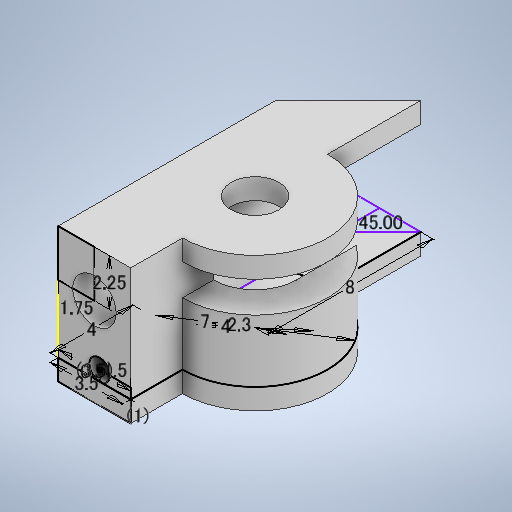
# Autodesk Inventor part: rod6.0
Saved by Autodesk Inventor 2025 (Build 290162000, 162)
## iProperties
Created: 2024-08-07
Part Number: rod6.0
Material: 一般
Document SubType Name: Modeling
Designer: Saigusa
Density: 1 g/cm^3
Appearance: 既定
Author: Saigusa
Autodesk Inventor part; units mm, degrees
ref_plane "YZ Plane" through (0, 0, 0) normal (1, 0, 0) x (0, 1, 0)
ref_plane "XZ Plane" through (0, 0, 0) normal (0, 1, 0) x (-1, 0, 0)
ref_plane "XY Plane" through (0, 0, 0) normal (0, 0, 1) x (1, 0, 0)
sketch "スケッチ1" plane through (0, 0, 0) normal (0, 1, 0) x (-1, 0, 0)
  circle A0 centre (0, 0) radius 1.15
  circle A1 centre (0, 0) radius 2
  circle A2 centre (0, 0) radius 3.5
  line L0 (0, 0) -> (0, 3.5)
  line L1 (2, 0) -> (-2, 0)
  line L2 (2, 0) -> (2, -2.8723)
  line L3 (-2, 0) -> (-2, -2.8723)
  line L4 (0, 2) -> (3.5, 2)
  line L5 (3.5, 2) -> (3.5, 6)
  line L6 (3.5, 6) -> (0, 6)
  line L7 (0, 6) -> (0, 2)
  line L8 (0, 6) -> (3.5, 6)
  line L9 (3.5, 6) -> (3.5, 0)
  line L10 (3.5, 0) -> (0, 0)
  line L11 (0, 0) -> (0, 6)
  line L12 (0, 0) -> (0, -8)
  line L13 (0, 0) -> (3.5, 0)
  line L14 (3.5, 0) -> (3.5, -8)
  line L15 (3.5, -8) -> (0, -8)
  line L16 (0, -8) -> (0, 0)
  line L17 (2, -2.8723) -> (2, -8)
  line L18 (0, -8) -> (3.5, -4.5)
  line L19 (0, -8) -> (4.9497, -8) construction
  point P0 (2, -6)
  point P1 (0, -3.5)
  dimension "d0" = 2.3
  dimension "d1" = 4
  dimension "d2" = 7
  dimension "d3" = 3.5
  dimension "d4" = 4
  dimension "d5" = 8
  dimension "d6" = 45
  constraints: 40 end point, 7 perpendicular, 7 point on circle, 6 parallel, 4 horizontal, 3 centre point, 3 coincident, 3 point on line, 2 vertical, 1 equal length
  measures "d0" diameter of A0
  measures "d1" diameter of A1
  measures "d2" diameter of A2
  measures "d3" distance of L6.end L5.end
  measures "d4" distance of L5.end L4.end
  measures "d5" distance of L10.end L12.end
  measures "d6" angle of L19 L18
extrude "押し出し1" add sketch "スケッチ1" along normal blind 3 contours A1 L3 A2 L0
extrude "押し出し2" add sketch "スケッチ1" along normal blind 4.5 contours L10 A2 L2 | A1 L4 A2 L10 | L0 A2 L4 | A2 L14 L18 L17 | A2 L4 L9 | L7 L6 L5 L4 A2
extrude "押し出し3" add sketch "スケッチ1" against normal blind 1 contours L1 A1 L12 A0 | A0 L0 A1 L1 | A0 L1 A1 L0 | L12 A1 L1 A0 | L2 A2 L12 A1 | L10 A2 L2 | A1 L4 A2 L10 | A1 L3 A2 L0 | L0 A2 L4 | L12 A2 L3 A1 | L17 L18 L12 A2 | A2 L14 L18 L17 | A2 L4 L9 | L7 L6 L5 L4 A2
sketch "スケッチ2" plane through (0, 4.5, 0) normal (0, 1, 0) x (1, 0, 0)
  circle A0 centre (0, 0) radius 1.15
  circle A1 centre (0, 0) radius 2
  circle A2 centre (0, 0) radius 3.5
  line L0 (0, -2) -> (0, -3.5) projected
  line L1 (-3.5, 4.5) -> (-3.5, -6) projected
  line L2 (0, -2) -> (-3.5, -2)
  line L3 (-3.5, -2) -> (-3.5, -6)
  line L4 (-3.5, -6) -> (0, -6)
  line L5 (0, -6) -> (0, -2)
  line L6 (0, -2) -> (-3.5, -2)
  line L7 (-3.5, -2) -> (-3.5, 8)
  line L8 (-3.5, 8) -> (0, 8)
  line L9 (0, 8) -> (0, -2)
  line L10 (0, 0) -> (-2, 0)
  line L11 (-2, 0) -> (-2, 8)
  line L12 (-2, 8) -> (0, 8)
  line L13 (0, 8) -> (0, 0)
  line L14 (0, 8) -> (-3.5, 4.5)
  line L15 (0, 8) -> (4.9497, 8) construction
  point P0 (0, 3.5)
  dimension "d14" = 4
  dimension "d15" = 7
  dimension "d13" = 2.3
  dimension "d16" = 3.5
  dimension "d17" = 4
  dimension "d18" = 3.5
  dimension "d19" = 10
  dimension "d20" = 2
  dimension "d21" = 8
  dimension "d22" = 135
  constraints: 28 end point, 6 parallel, 4 horizontal, 3 coincident, 3 perpendicular, 1 centre point, 1 equal length, 1 vertical alignment, 3 other
  measures "d13" diameter of A0
  measures "d16" distance of L4.end L1.end
  measures "d17" distance of L1.end L2.end
  measures "d18" distance of L7.end L8.end
  measures "d19" distance of L6.end L7.end
  measures "d20" distance of L11.end L12.end
  measures "d21" distance of L10.end L11.end
  measures "d22" angle of L14 L15
extrude "押し出し4" add sketch "スケッチ2" along normal blind 1 contours A0 L9 A1 | A0 L10 A1 L9 | L9 A1 L10 A0 | L9 A2 L0 A1 | A1 L11 A2 L9 | L2 A2 L11 A1 | L0 A2 L2 | A2 L11 L14 L9 | L5 L4 L1 L2 A2 | L2 L1 A2 | A2 L1 L14 L11
sketch "スケッチ3" plane through (-3.5, -1, 6) normal (0, 0, 1) x (1, 0, 0)
  line L0 (0, 0) -> (0, 6.5) projected
  line L1 (0, 0) -> (3.5, 0)
  line L2 (3.5, 0) -> (3.5, 1)
  line L3 (3.5, 1) -> (0, 1)
  line L4 (0, 1) -> (0, 0)
  line L5 (3.5, 1) -> (2, 1)
  line L6 (2, 1) -> (2, 1.5)
  line L7 (2, 1.5) -> (3.5, 1.5)
  line L8 (3.5, 1.5) -> (3.5, 1)
  circle A0 centre (2, 1.5) radius 0.5
  line L9 (0, 6.5) -> (1.75, 6.5)
  line L10 (1.75, 6.5) -> (1.75, 4.25)
  line L11 (1.75, 4.25) -> (0, 4.25)
  line L12 (0, 4.25) -> (0, 6.5)
  dimension "d25" = 3.5
  dimension "d26" = 1
  dimension "d27" = 1.5
  dimension "d28" = 0.5
  dimension "d29" = 1.75
  dimension "d30" = 2.25
  constraints: 24 end point, 6 parallel, 3 horizontal, 3 perpendicular, 1 coincident, 1 vertical alignment, 2 other
  measures "d25" distance of L3.end L2.end
  measures "d26" distance of L2.end L1.end
  measures "d27" distance of L6.end L7.end
  measures "d28" distance of L5.end L6.end
  measures "d29" distance of L10.end L11.end
  measures "d30" distance of L9.end L10.end
extrude "押し出し5" cut sketch "スケッチ3" against normal blind 6 contours A0 L7 L6 | L6 L7 A0
hole "穴1" at (-1.75, 3.25, 6) direction (0, 0, -1) diameter 2.1 depth 4
